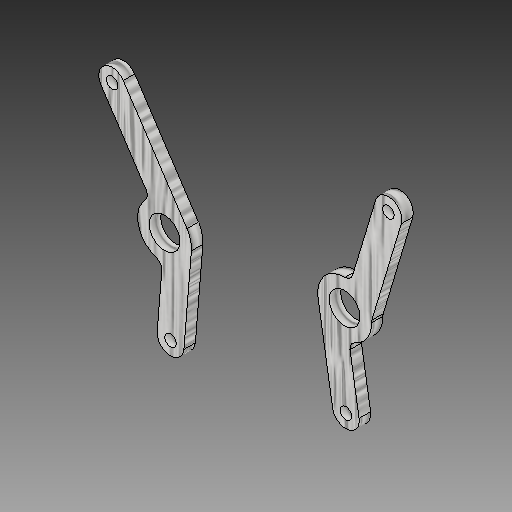
# Autodesk Inventor part: サス軸抑え外
Saved by Autodesk Inventor 2019 (Build 230136000, 136)
## iProperties
Created: 2019-11-12
Part Number: サス軸抑え外
Material: アルミニウム 7075
Document SubType Name: Modeling
Designer: tanjihayato
Density: 2.81 g/cm^3
Appearance: サテン - ブラシ仕上げ 重厚
Mass: 7.14611 g
Surface Area: 27.7053 cm^2
Volume: 2.5431 cm^3
Author: tanjihayato
Autodesk Inventor part; units mm, degrees
ref_plane "YZ Plane" through (0, 0, 0) normal (1, 0, 0) x (0, 1, 0)
ref_plane "XZ Plane" through (0, 0, 0) normal (0, 1, 0) x (-1, 0, 0)
ref_plane "XY Plane" through (0, 0, 0) normal (0, 0, 1) x (1, 0, 0)
sketch "スケッチ1" plane through (0, 0, 0) normal (0, 0, 1) x (1, 0, 0)
  circle A0 centre (0, 0) radius 20.55 construction
  circle A1 centre (-21.6908, -16.4118) radius 19.1 construction
  circle A2 centre (25.3202, -9.9362) radius 19.1 construction
  circle A3 centre (-50.601, 30.8143) radius 1.5
  circle A4 centre (5.9362, 53.5882) radius 1.5
  circle A5 centre (27.3908, 10.6821) radius 1.5
  circle A6 centre (-42.8914, 18.3887) radius 1.5
  circle A7 centre (-21.6908, -16.4118) radius 4.025
  circle A8 centre (25.3202, -9.9362) radius 4.025
  circle A9 centre (0, 0) radius 4
  line L0 (-17.8785, -18.8026) -> (-30.4168, -38.7963) construction
  arc A10 (-17.8785, -18.8026) -> (-19.2493, -12.6317) centre (-21.6908, -16.4118) ccw construction
  line L1 (-19.2493, -12.6317) -> (-39.0737, 0.1727) construction
  line L2 (37.1409, -30.8522) -> (21.8866, -12.8448) construction
  arc A11 (22.3659, -6.5417) -> (21.8866, -12.8448) centre (25.3202, -9.9362) ccw construction
  line L3 (22.3659, -6.5417) -> (40.1678, 8.9519) construction
  line L4 (-21.6908, -16.4118) -> (-99.9742, 13.5882) construction
  line L5 (-105.5257, -16.4118) -> (-21.6908, -16.4118) construction
  line L6 (-21.6908, -16.4118) -> (-101.7113, -41.4118) construction
  line L7 (25.3202, -9.9362) -> (102.5386, -46.4118) construction
  line L8 (110.4743, -16.4118) -> (25.3202, -9.9362) construction
  line L9 (25.3202, -9.9362) -> (108.6869, 8.5882) construction
  line L10 (-18.0583, -13.7557) -> (-31.9879, 5.2949) construction
  line L11 (-17.339, -17.5569) -> (-24.5367, -44.9106) construction
  line L12 (21.5077, -7.5456) -> (34.045, 12.4488) construction
  line L13 (21.0739, -11.4259) -> (31.6059, -41.446) construction
  arc A12 (-24.6176, -40.3201) -> (-19.5065, -44.4166) centre (-20.132, -39.9603) ccw
  circle A13 centre (-20.132, -39.9603) radius 3 construction
  arc A14 (-38.9879, 7.9907) -> (-39.3359, 8.5262) centre (-35.3982, 10.7044) ccw construction
  circle A15 centre (-35.3982, 10.7044) radius 3 construction
  arc A16 (-31.9879, 5.2949) -> (-33.8465, 6.7744) centre (-35.6204, 2.6388) ccw construction
  circle A17 centre (-41.5152, -3.6073) radius 1.5
  line L14 (-33.8465, 6.7744) -> (-56.066, 16.3055) construction
  line L15 (-41.3386, 0.8892) -> (-72.6317, 2.1181) construction
  circle A18 centre (-42.8914, 18.3887) radius 3 construction
  circle A19 centre (-35.3982, 10.7044) radius 1.5
  circle A20 centre (36.7736, 17.5344) radius 1.5
  arc A21 (40.7942, 15.5132) -> (40.1934, 20.4593) centre (36.7736, 17.5344) ccw
  circle A22 centre (25.6508, -33.5339) radius 1.5
  arc A23 (26.2763, -37.9902) -> (30.1508, -33.5178) centre (25.6508, -33.5339) ccw
  circle A24 centre (36.7736, 17.5344) radius 3 construction
  circle A25 centre (25.6508, -33.5339) radius 3 construction
  arc A26 (36.6836, 14.4025) -> (34.045, 12.4488) centre (37.8575, 10.0583) ccw construction
  line L16 (36.6836, 14.4025) -> (64.1968, 21.8369) construction
  line L17 (43.2599, 10.0553) -> (82.9273, 8.8396) construction
  circle A27 centre (27.3908, 10.6821) radius 3 construction
  circle A28 centre (-21.6908, -16.4118) radius 7.025 construction
  circle A29 centre (25.3202, -9.9362) radius 7.025 construction
  arc A30 (40.8593, 15.6483) -> (30.1508, -33.5178) centre (146.4685, -33.1029) ccw
  arc A31 (-24.6176, -40.3201) -> (-39.1827, 8.2484) centre (-145.1158, -49.988) ccw
  arc A32 (-52.2824, 34.9884) -> (-54.1907, 28.1005) centre (-50.601, 30.8143) ccw
  arc A33 (9.356, 56.5132) -> (4.2549, 57.7623) centre (5.9362, 53.5882) ccw
  line L18 (-39.1827, 8.2484) -> (-54.1907, 28.1005)
  line L19 (-52.2824, 34.9884) -> (4.2549, 57.7623)
  line L20 (9.356, 56.5132) -> (40.1934, 20.4593)
  line L21 (-19.5065, -44.4166) -> (26.2763, -37.9902)
  circle A34 centre (-20.132, -39.9603) radius 1.5
  line L22 (-23.8868, -42.4405) -> (-17.339, -17.5569)
  arc A35 (-17.339, -17.5569) -> (-18.0583, -13.7557) centre (-21.6908, -16.4118) ccw
  line L23 (-18.0583, -13.7557) -> (-31.9879, 5.2949)
  arc A36 (-31.9879, 5.2949) -> (-33.8465, 6.7744) centre (-35.6204, 2.6388) ccw
  line L24 (-33.8465, 6.7744) -> (-40.0946, 9.4545)
  line L25 (40.7974, 15.5141) -> (36.6836, 14.4025)
  arc A37 (36.6836, 14.4025) -> (34.045, 12.4488) centre (37.8575, 10.0583) ccw
  line L26 (34.045, 12.4488) -> (21.5077, -7.5456)
  arc A38 (21.5077, -7.5456) -> (21.0739, -11.4259) centre (25.3202, -9.9362) ccw
  line L27 (21.0739, -11.4259) -> (29.592, -35.7057)
  dimension "d0" = 8.05
  dimension "d1" = 8.05
  dimension "d2" = 8
  dimension "d3" = 20.968
  dimension "d4" = 20.968
  dimension "d5" = 17.35
  dimension "d6" = 17.35
  dimension "d7" = 16.877
  dimension "d8" = 16.877
  dimension "d9" = 20.936
  dimension "d10" = 20.936
  dimension "d11" = 9
  dimension "d12" = 6
  dimension "d13" = 9
  dimension "d14" = 6
  dimension "d15" = 9
  dimension "d16" = 20.968
  dimension "d17" = 20.968
  dimension "d18" = 6
  dimension "d19" = 3
  dimension "d20" = 3
  dimension "d21" = 9
  dimension "d22" = 3
  dimension "d23" = 9
  dimension "d24" = 6
  dimension "d25" = 6
  dimension "d26" = 9
  dimension "d27" = 16.877
  dimension "d28" = 3
  dimension "d29" = 3
  dimension "d30" = 9
  dimension "d31" = 9
  dimension "d32" = 3
  constraints: 56 end point, 40 point on circle, 39 centre point, 31 tangent, 14 coincident, 6 point on line, 2 equal length, 1 collinear, 1 concentric
  measures "d0" diameter of A7
  measures "d1" diameter of A8
  measures "d2" diameter of A9
  measures "d3" angle of L5 L4
  measures "d4" angle of L1 L10
  measures "d5" angle of L5 L6
  measures "d6" angle of L0 L11
  measures "d7" angle of L8 L9
  measures "d8" angle of L12 L3
  measures "d9" angle of L8 L7
  measures "d10" angle of L13 L2
  measures "d11" diameter of A12
  measures "d12" diameter of A13
  measures "d13" diameter of A14
  measures "d14" diameter of A15
  measures "d15" diameter of A16
  measures "d17" angle of L15 L14
  measures "d18" diameter of A18
  measures "d19" diameter of A19
  measures "d20" diameter of A20
  measures "d21" diameter of A21
  measures "d22" diameter of A22
  measures "d23" diameter of A23
  measures "d24" diameter of A24
  measures "d25" diameter of A25
  measures "d26" diameter of A26
  measures "d27" angle of L16 L17
  measures "d28" radial gap between concentric circles of A7 A28
  measures "d29" radial gap between concentric circles of A8 A29
  measures "d30" diameter of A32
  measures "d31" diameter of A33
  measures "d32" diameter of A34
sketch "スケッチ2" plane through (0, 0, 0) normal (0, 0, 1) x (1, 0, 0)
  circle A0 centre (-35.3982, 10.7044) radius 1.5 projected
  circle A1 centre (-21.6908, -16.4118) radius 4.025 projected
  circle A2 centre (-20.132, -39.9603) radius 1.5 projected
  circle A3 centre (25.6508, -33.5339) radius 1.5 projected
  circle A4 centre (25.3202, -9.9362) radius 4.025 projected
  circle A5 centre (36.7736, 17.5344) radius 1.5 projected
  circle A6 centre (-35.3982, 10.7044) radius 4.5
  circle A7 centre (-21.6908, -16.4118) radius 7.025
  circle A8 centre (-20.132, -39.9603) radius 4.5
  circle A9 centre (36.7736, 17.5344) radius 4.5
  circle A10 centre (25.3202, -9.9362) radius 7.025
  circle A11 centre (25.6508, -33.5339) radius 4.5
  line L0 (-31.5648, 13.0613) -> (-15.7064, -12.7325)
  line L1 (-14.6718, -16.7004) -> (-15.6358, -40.1451)
  line L2 (-24.5646, -40.7362) -> (-28.6106, -17.6231)
  line L3 (-39.5691, 9.015) -> (-28.202, -19.0491)
  line L4 (41.059, 16.1613) -> (32.0102, -12.0797)
  line L5 (32.7821, 19.6122) -> (19.0889, -6.6924)
  line L6 (18.3467, -10.7856) -> (21.1838, -34.078)
  line L7 (30.1313, -33.9526) -> (32.3147, -10.5899)
  point P0 (0, 0)
  dimension "d33" = 3
  dimension "d34" = 3
  dimension "d35" = 3
  dimension "d36" = 3
  dimension "d37" = 3
  dimension "d38" = 3
  constraints: 16 end point, 16 point on circle, 16 tangent, 6 centre point
  measures "d33" radial gap between concentric circles of A0 A6
  measures "d34" radial gap between concentric circles of A1 A7
  measures "d35" radial gap between concentric circles of A2 A8
  measures "d36" radial gap between concentric circles of A5 A9
  measures "d37" radial gap between concentric circles of A4 A10
  measures "d38" radial gap between concentric circles of A3 A11
extrude "押し出し1" add sketch "スケッチ2" along normal blind 3
sketch "スケッチ3" plane through (0, 0, 0) normal (0, 0, -1) x (-1, 0, 0)
  circle A0 centre (-25.3202, -9.9362) radius 4.025 projected
  circle A1 centre (-25.6508, -33.5339) radius 1.5 projected
  circle A2 centre (-36.7736, 17.5344) radius 1.5 projected
  arc A3 (-32.7821, 19.6122) -> (-41.059, 16.1613) centre (-36.7736, 17.5344) ccw projected
  line L0 (-32.2435, -11.3514) -> (-41.059, 16.1613) projected
  line L1 (-30.1313, -33.9526) -> (-32.2435, -11.3514) projected
  arc A4 (-30.1313, -33.9526) -> (-21.1838, -34.078) centre (-25.6508, -33.5339) ccw projected
  line L2 (-18.3467, -10.7856) -> (-21.1838, -34.078) projected
  arc A5 (-18.3467, -10.7856) -> (-19.0889, -6.6924) centre (-25.3202, -9.9362) ccw projected
  line L3 (-32.7821, 19.6122) -> (-19.0889, -6.6924) projected
  circle A6 centre (21.6908, -16.4118) radius 4.025 projected
  circle A7 centre (35.3982, 10.7044) radius 1.5 projected
  circle A8 centre (20.132, -39.9603) radius 1.5 projected
  arc A9 (15.6358, -40.1451) -> (24.5646, -40.7362) centre (20.132, -39.9603) ccw projected
  line L4 (28.482, -18.3578) -> (24.5646, -40.7362) projected
  line L5 (39.5691, 9.015) -> (28.482, -18.3578) projected
  arc A10 (39.5691, 9.015) -> (31.5648, 13.0613) centre (35.3982, 10.7044) ccw projected
  line L6 (15.7064, -12.7325) -> (31.5648, 13.0613) projected
  arc A11 (15.7064, -12.7325) -> (14.6718, -16.7004) centre (21.6908, -16.4118) ccw projected
  line L7 (15.6358, -40.1451) -> (14.6718, -16.7004) projected
  circle A12 centre (-25.3202, -9.9362) radius 6
  circle A13 centre (21.6908, -16.4118) radius 6
  point P0 (0, 0)
  dimension "d41" = 12
  dimension "d42" = 12
  constraints: 2 centre point, 2 coincident
  measures "d41" diameter of A12
  measures "d42" diameter of A13
sketch "スケッチ4" plane through (0, 0, 3) normal (0, 0, 1) x (1, 0, 0)
  circle A0 centre (27.3908, 10.6821) radius 3 construction
  circle A1 centre (27.3908, 10.6821) radius 3.5 construction
  circle A2 centre (36.7736, 17.5344) radius 1.5 projected
  circle A3 centre (25.6508, -33.5339) radius 1.5 projected
  circle A4 centre (25.3202, -9.9362) radius 4.025 projected
  arc A5 (19.0889, -6.6924) -> (18.3467, -10.7856) centre (25.3202, -9.9362) ccw projected
  line L0 (18.3467, -10.7856) -> (21.1838, -34.078) projected
  arc A6 (21.1838, -34.078) -> (30.1313, -33.9526) centre (25.6508, -33.5339) ccw projected
  line L1 (30.1313, -33.9526) -> (32.2435, -11.3514) projected
  line L2 (32.2435, -11.3514) -> (41.059, 16.1613) projected
  arc A7 (41.059, 16.1613) -> (32.7821, 19.6122) centre (36.7736, 17.5344) ccw projected
  line L3 (32.7821, 19.6122) -> (19.0889, -6.6924) projected
  arc A8 (32.7821, 19.6122) -> (32.2798, 17.7701) centre (36.7736, 17.5344) ccw
  arc A9 (20.9133, -4.4653) -> (19.0889, -6.6924) centre (25.3202, -9.9362) ccw
  arc A10 (20.9133, -4.4653) -> (32.2798, 17.7701) centre (1.7102, 19.374) ccw
  point P0 (0, 0)
  dimension "d45" = 7
  dimension "d48" = 4.5
  constraints: 6 point on circle, 4 centre point, 3 coincident, 3 tangent, 2 point on line, 1 concentric
  measures "d45" diameter of A1
  measures "d48" radius of A8
extrude "押し出し4" cut sketch "スケッチ4" against normal blind 3 contours L3 A8 A10 A9
sketch "スケッチ5" plane through (0, 0, 3) normal (0, 0, 1) x (1, 0, 0)
  circle A0 centre (-20.132, -39.9603) radius 1.5 projected
  circle A1 centre (-35.3982, 10.7044) radius 1.5 projected
  circle A2 centre (-21.6908, -16.4118) radius 4.025 projected
  arc A3 (-14.6718, -16.7004) -> (-15.7064, -12.7325) centre (-21.6908, -16.4118) ccw projected
  line L0 (-15.7064, -12.7325) -> (-31.5648, 13.0613) projected
  arc A4 (-31.5648, 13.0613) -> (-39.5691, 9.015) centre (-35.3982, 10.7044) ccw projected
  line L1 (-39.5691, 9.015) -> (-28.482, -18.3578) projected
  line L2 (-28.482, -18.3578) -> (-24.5646, -40.7362) projected
  arc A5 (-24.5646, -40.7362) -> (-15.6358, -40.1451) centre (-20.132, -39.9603) ccw projected
  line L3 (-15.6358, -40.1451) -> (-14.6718, -16.7004) projected
  arc A6 (41.059, 16.1613) -> (32.2798, 17.7701) centre (36.7736, 17.5344) ccw projected
  arc A7 (20.9133, -4.4653) -> (32.2798, 17.7701) centre (1.7102, 19.374) ccw projected
  arc A8 (20.9133, -4.4653) -> (18.3467, -10.7856) centre (25.3202, -9.9362) ccw projected
  line L4 (18.3467, -10.7856) -> (21.1838, -34.078) projected
  arc A9 (21.1838, -34.078) -> (30.1313, -33.9526) centre (25.6508, -33.5339) ccw projected
  line L5 (30.1313, -33.9526) -> (32.2435, -11.3514) projected
  line L6 (32.2435, -11.3514) -> (41.059, 16.1613) projected
  circle A10 centre (25.3202, -9.9362) radius 4.025 projected
  circle A11 centre (25.6508, -33.5339) radius 1.5 projected
  circle A12 centre (36.7736, 17.5344) radius 1.5 projected
  arc A13 (-32.4789, 12.6351) -> (-38.3175, 8.7737) centre (-35.3982, 10.7044) ccw
  arc A14 (-23.6197, -39.6672) -> (-16.6443, -40.2533) centre (-20.132, -39.9603) ccw
  arc A15 (22.1977, -34.1051) -> (29.1039, -32.9627) centre (25.6508, -33.5339) ccw
  arc A16 (40.1258, 16.528) -> (33.4214, 18.5407) centre (36.7736, 17.5344) ccw
  line L7 (-38.3175, 8.7737) -> (-25.5452, -10.5386)
  line L8 (-32.4789, 12.6351) -> (-15.8314, -12.5366)
  line L9 (-16.6443, -40.2533) -> (-14.6905, -17)
  line L10 (-23.6197, -39.6672) -> (-22.2541, -23.4142)
  arc A17 (-25.5452, -10.5386) -> (-22.2541, -23.4142) centre (-21.6908, -16.4118) ccw
  arc A18 (-14.6905, -17) -> (-15.8314, -12.5366) centre (-21.6908, -16.4118) ccw
  line L11 (40.1258, 16.528) -> (32.3281, -9.446)
  line L12 (33.4214, 18.5407) -> (26.9255, -3.097)
  line L13 (22.1977, -34.1051) -> (18.3894, -11.0827)
  line L14 (29.1039, -32.9627) -> (26.442, -16.871)
  arc A19 (20.9133, -4.4653) -> (32.2798, 17.7701) centre (1.7102, 19.374) ccw projected
  arc A20 (26.9255, -3.097) -> (18.3894, -11.0827) centre (25.3202, -9.9362) ccw
  arc A21 (26.442, -16.871) -> (32.3281, -9.446) centre (25.3202, -9.9362) ccw
  point P0 (0, 0)
  dimension "d52" = 7
  dimension "d53" = 7
  dimension "d54" = 7
  dimension "d55" = 7
  dimension "d56" = 3
  dimension "d57" = 3
  constraints: 16 end point, 16 point on circle, 12 tangent, 8 centre point, 6 coincident, 4 parallel, 2 concentric
  measures "d52" diameter of A13
  measures "d53" diameter of A14
  measures "d54" diameter of A15
  measures "d55" diameter of A16
  measures "d56" radial gap between concentric circles of A18 A2
  measures "d57" radial gap between concentric circles of A21 A10
extrude "押し出し5" cut sketch "スケッチ5" against normal blind 10 contours L3 A5 L2 L1 A4 L0 A18 L8 A13 L7 A17 L10 A14 L9 | L6 L5 A9 L4 A20 L13 A15 L14 A21 L11 A16 L12 A7 A6 | L12 A20 A7
fillet "フィレット1" radius 2 5 edges at (-25.5452, -10.5386, 1.5) (-22.2541, -23.4142, 1.5) (26.9255, -3.097, 1.5) (26.442, -16.871, 1.5) (32.3281, -9.446, 1.5)
equation "\"d4\" = d3"
equation "\"d6\" = d5"
equation "\"d8\" = d7"
equation "\"d10\" = d9"
equation "\"d16\" = d3"
equation "\"d17\" = d3"
equation "\"d27\" = d7"
